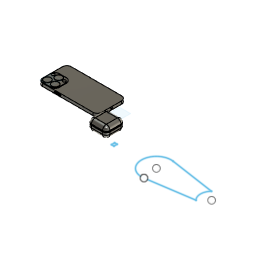
Galaxy Buds v3 (Autodesk Fusion 360 design; units mm, degrees)
Autodesk Fusion 360 part; units mm, degrees
note: some values were not read from the file. Chosen so that the rebuilt part matches the saved one: which bodies a step acts on; which face or edge a step refers to; that a step has no effect.
sketch "Sketch1" plane through (0, 0, 0) normal (0, 0, 1) x (1, 0, 0)
  line L0 (0, 0) -> (50.2, 0)
  line L1 (50.2, 0) -> (50.2, 50)
  line L2 (50.2, 50) -> (0, 50)
  line L3 (0, 50) -> (0, 0)
  dimension "d1" = 50.2
  dimension "d2" = 50
  constraint horizontal L0
  constraint vertical L1
  constraint horizontal L2
  constraint vertical L3
  constraint coincident L0.start L3.end
  measures "d1" distance of L0.start L0.end
  measures "d2" distance of L0.start L2.end
extrude "Extrude1" add sketch "Sketch1" along normal blind 27.88 makes body 1
fillet "Fillet1" radius 10 12 edges at (50.2, 0, 13.94) (25.1, 0, 27.88) (50.2, 25, 27.88) (50.2, 50, 13.94) (50.2, 25, 0) (25.1, 0, 0) (0, 0, 13.94) (0, 25, 27.88) (0, 50, 13.94) (0, 25, 0) (25.1, 50, 0) (25.1, 50, 27.88) on bodies 1
form "Form1" [no effect]
sketch "Sketch2" plane through (0, 0, 0) normal (0, 0, 1) x (1, 0, 0)
  line L0 (0, -10) -> (48, -10)
  line L1 (48, -10) -> (48, -58)
  line L2 (48, -58) -> (0, -58)
  line L3 (0, -58) -> (0, -10)
  dimension "d7" = 48
  dimension "d8" = 48
  constraint horizontal L0
  constraint vertical L1
  constraint horizontal L2
  constraint vertical L3
  measures "d7" distance of L0.start L0.end
  measures "d8" distance of L0.start L2.end
sketch "Sketch3" plane through (0, 0, 0) normal (0, 0, 1) x (1, 0, 0)
  line L0 (150, 0) -> (98.8, 0)
  line L1 (98.8, 0) -> (98.8, 51)
  line L2 (98.8, 51) -> (150, 51)
  line L3 (150, 51) -> (150, 0)
  dimension "d11" = 51.2
  dimension "d12" = 51
  constraint horizontal L0
  constraint vertical L1
  constraint horizontal L2
  constraint vertical L3
  measures "d11" distance of L0.start L0.end
  measures "d12" distance of L0.start L2.end
extrude "Extrude3" add sketch "Sketch3" along normal blind 1 separate body makes body 2
move_body "Move1" bodies 2 to x (1, 0, 0) y (0, 1, 0) z (0, 0, 1) at (-99, 0, 15)
split "Split1" by plane through (-99, 0, 16) normal (0, 0, 1) bodies 1 makes body 3 at (30.1333, 20, 27.88)
move_body "Move2" bodies 3 to x (1, 0, 0) y (0, 1, 0) z (0, 0, 1) at (0, 0, 1)
move_body "Move3" bodies 2 to x (1, 0, 0) y (0, 1, 0) z (0, 0, 1) at (0, 20, 0)
move_body "Move4" bodies 2 to x (1, 0, 0) y (0, 1, 0) z (0, 0, 1) at (0, 100, 0)
sketch "Sketch4" plane through (0, 0, 0) normal (0, 0, 1) x (1, 0, 0)
  line L0 (0, 0) -> (-49.2, 0)
  line L1 (-49.2, 0) -> (-49.2, -49)
  line L2 (-49.2, -49) -> (0, -49)
  line L3 (0, -49) -> (0, 0)
  dimension "d15" = 49.2
  dimension "d16" = 49
  constraint horizontal L0
  constraint vertical L1
  constraint horizontal L2
  constraint vertical L3
  constraint coincident L0.start L3.end
  measures "d15" distance of L0.start L0.end
  measures "d16" distance of L0.start L2.end
extrude "Extrude4" add sketch "Sketch4" along normal blind 1 separate body makes body 4
move_body "Move5" bodies 4 to x (1, 0, 0) y (0, 1, 0) z (0, 0, 1) at (-17, 0, 0)
sketch "Sketch5" plane through (0, 0, 0) normal (0, 1, 0) x (1, 0, 0)
sketch "Sketch6" plane through (0, 0, 1) normal (0, 0, 1) x (-1, 0, 0)
  line L0 (17, 49) -> (17, 0)
  line L1 (17, 0) -> (66.2, 0)
  line L2 (66.2, 0) -> (66.2, 49)
  line L3 (66.2, 49) -> (17, 49)
sketch "Sketch7" plane through (0, 0, 0) normal (0, 0, 1) x (1, 0, 0)
  line L0 (-24.854, -48.854) -> (-17, -48.854)
  line L1 (-17, -48.854) -> (-17, -41)
  line L2 (-17, -41) -> (-24.854, -48.854)
  line L3 (-16.927, -7.781) -> (-16.927, 0.073)
  line L4 (-24.781, 0.073) -> (-16.927, -7.781)
  line L5 (-16.927, 0.073) -> (-24.781, 0.073)
  line L6 (-81.35, 0.006) -> (-89.204, 0.006)
  line L7 (-89.204, -7.848) -> (-81.35, 0.006)
  line L8 (-89.204, 0.006) -> (-89.204, -7.848)
  line L9 (-66.277, -41.067) -> (-66.277, -48.921)
  line L10 (-66.277, -48.921) -> (-58.423, -48.921)
  line L11 (-58.423, -48.921) -> (-66.277, -41.067)
  dimension "d20" = 7.854
  dimension "d21" = 7.854
  dimension "d22" = 7.854
  dimension "d23" = 7.854
  constraint horizontal L0
  constraint vertical L1
  measures "d20" distance of L1.end L0.end
  measures "d21" distance of L4.start L3.end
  measures "d22" distance of L7.start L6.end
  measures "d23" distance of L9.end L10.end
extrude "Extrude5" add sketch "Sketch7" along normal blind 1 separate body contours L6 L7 L8 makes body 5
move_body "Move6" bodies 5 to x (1, 0, 0) y (0, 1, 0) z (0, 0, 1) at (0, 12, 0)
move_body "Move7" bodies 5 to x (1, 0, 0) y (0, 1, 0) z (0, 0, 1) at (23, -12, 0)
split "Split2" by bodies 5 bodies 4 makes body 6 at (-30.7853, -16.3333, 0)
move_body "Move8" bodies 4 to x (1, 0, 0) y (0, 1, 0) z (0, 0, 1) at (0, 9, 0)
extrude "Extrude6" add 1 faces at (-63.5853, 6.3853, 1) along direction (0, 0, 1) blind 1 on bodies 4 bodies 4
move_body "Move9" bodies 4 to x (1, 0, 0) y (0, 1, 0) z (0, 0, 1) at (0, -9, 0)
move_body "Move10" bodies 2 to x (1, 0, 0) y (0, 1, 0) z (0, 0, 1) at (0, -121, 3)
split "Split3" by plane through (-99, -1, 19) normal (0, 0, 1) bodies 3 makes body 7 at (30.1333, 20, 28.88)
move_body "Move11" bodies 3 2 to x (1, 0, 0) y (0, 1, 0) z (0, 0, 1) at (0, 60, 0)
move_body "Move12" bodies 3 to x (1, 0, 0) y (0, 1, 0) z (0, 0, 1) at (137, 0, -11)
scale "Scale1" factor 0.99 about (187.2, 70, 6) bodies 3
move_body "Move13" bodies 3 to x (1, 0, 0) y (0, 1, 0) z (0, 0, 1) at (-138, -60, 10)
move_body "Move14" bodies 3 to x (1, 0, 0) y (0, 1, 0) z (0, 0, 1) at (0.75, 0, 0)
move_body "Move15" bodies 3 to x (1, 0, 0) y (0, 1, 0) z (0, 0, 1) at (0, 0.3, 0)
sketch "Sketch8" plane through (0, 0, 17.98) normal (0, 0, 1) x (-1, 0, 0)
  arc A0 (-40.05, -0.4007) -> (-49.9493, -10.3) centre (-40.05, -10.3) ccw
  line L0 (-49.9493, -10.3) -> (-49.9493, -40)
  arc A1 (-49.9493, -40) -> (-40.05, -49.8993) centre (-40.05, -40) ccw
  line L1 (-40.05, -49.8993) -> (-10.152, -49.8993)
  arc A2 (-10.152, -49.8993) -> (-0.2527, -40) centre (-10.152, -40) ccw
  line L2 (-0.2527, -40) -> (-0.2527, -10.3)
  arc A3 (-0.2527, -10.3) -> (-10.152, -0.4007) centre (-10.152, -10.3) ccw
  line L3 (-10.152, -0.4007) -> (-40.05, -0.4007)
extrude "Extrude7" add sketch "Sketch8" along normal blind 1 bodies 3
move_body "Move16" bodies 2 to x (1, 0, 0) y (0, 1, 0) z (0, 0, 1) at (-94, 0, 0)
sketch "Sketch9" plane through (0, 0, 0) normal (0, 0, 1) x (1, 0, 0)
  line L0 (65, -30) -> (58.35, -30)
  line L1 (58.35, -30) -> (58.35, -21.6)
  line L2 (58.35, -21.6) -> (65, -21.6)
  line L3 (65, -21.6) -> (65, -30)
  dimension "d31" = 6.65
  dimension "d32" = 8.4
  constraint horizontal L0
  constraint vertical L1
  constraint horizontal L2
  constraint vertical L3
  measures "d31" distance of L0.start L0.end
  measures "d32" distance of L0.start L2.end
sketch "Sketch10" plane through (0, 0, 0) normal (1, 0, 0) x (0, 1, 0)
sketch "Sketch11" plane through (0, 0, 0) normal (0, 1, 0) x (1, 0, 0)
  line L0 (44.2, 10) -> (47.545, 10)
  line L1 (44.2, 10) -> (40.855, 10)
  line L2 (44.2, 12.6) -> (40.855, 12.6)
  line L3 (44.2, 12.6) -> (47.545, 12.6)
  arc A0 (47.545, 10) -> (47.545, 12.6) centre (46.9842, 11.3) ccw
  arc A1 (40.855, 12.6) -> (40.855, 10) centre (41.4158, 11.3) ccw
  dimension "d35" = 3.345
  dimension "d36" = 3.345
  dimension "d37" = 3.345
  dimension "d38" = 3.345
  measures "d35" distance of L0.start L0.end
  measures "d36" distance of L0.start L1.end
  measures "d37" distance of L2.start L2.end
  measures "d38" distance of L2.start L3.end
extrude "Extrude8" add sketch "Sketch11" along normal blind 6.65 separate body makes body 8
move_body "Move17" bodies 8 to x (1, 0, 0) y (0, 1, 0) z (0, 0, 1) at (-18, 44, 23)
move_body "Move18" bodies 8 to x (1, 0, 0) y (0, 1, 0) z (0, 0, 1) at (-0.0267, -0.5, -0.4993)
sketch "Sketch12" plane through (0, 0, 0) normal (0, 1, 0) x (1, 0, 0)
split "Split4" by bodies 8 bodies 1 makes body 9 at (20.0667, 16.6667, 16)
move_body "Move19" bodies 8 to x (1, 0, 0) y (0, 1, 0) z (0, 0, 1) at (0, 19, 0)
move_body "Move20" bodies 1 to x (1, 0, 0) y (0, 1, 0) z (0, 0, 1) at (0, 69, 0)
delete_body "RemoveBody1" bodies 1
sketch "Sketch13" plane through (0, 0, 0) normal (0, 1, 0) x (1, 0, 0)
sketch "Sketch14" plane through (0, 0, 0) normal (0, 0, 1) x (1, 0, 0)
  line L0 (-23, 13) -> (-183.6, 13)
  line L1 (-183.6, 13) -> (-183.6, 90.6)
  line L2 (-183.6, 90.6) -> (-23, 90.6)
  line L3 (-23, 90.6) -> (-23, 13)
  dimension "d41" = 160.6
  dimension "d42" = 77.6
  constraint horizontal L0
  constraint vertical L1
  constraint horizontal L2
  constraint vertical L3
  measures "d41" distance of L0.start L0.end
  measures "d42" distance of L0.start L2.end
extrude "Extrude9" add sketch "Sketch14" along normal blind 7.85 separate body makes body 10
fillet "Fillet2" radius 12 4 edges at (-23, 90.6, 3.925) (-23, 13, 3.925) (-183.6, 90.6, 3.925) (-183.6, 13, 3.925) on bodies 10
sketch "Sketch15" plane through (0, 0, 0) normal (0, 0, 1) x (1, 0, 0)
sketch "Sketch16" plane through (0, 0, 0) normal (0, 0, 1) x (1, 0, 0)
  line L0 (0, -25) -> (-30, -25)
  line L1 (-30, -25) -> (-30, 5)
  line L2 (-30, 5) -> (0, 5)
  line L3 (0, 5) -> (0, -25)
  dimension "d47" = 30
  dimension "d48" = 30
  constraint horizontal L0
  constraint vertical L1
  constraint horizontal L2
  constraint vertical L3
  measures "d47" distance of L0.start L0.end
  measures "d48" distance of L0.start L2.end
extrude "Extrude10" add sketch "Sketch16" along normal blind 1 separate body makes body 11
move_body "Move21" bodies 11 to x (1, 0, 0) y (0, 1, 0) z (0, 0, 1) at (-145, 45, 15)
move_body "Move22" bodies 11 to x (1, 0, 0) y (0, 1, 0) z (0, 0, 1) at (0, -8, -3)
move_body "Move23" bodies 11 to x (1, 0, 0) y (0, 1, 0) z (0, 0, 1) at (0, 0, -4)
move_body "Move24" bodies 11 to x (1, 0, 0) y (0, 1, 0) z (0, 0, 1) at (-7, 3, 0)
sketch "Sketch17" plane through (0, 0, 9) normal (0, 0, 1) x (-1, 0, 0)
  line L0 (152, -45) -> (182, -45)
  line L1 (182, -45) -> (182, -15)
  line L2 (182, -15) -> (152, -15)
  line L3 (152, -15) -> (152, -45)
move_body "Move25" bodies 11 to x (1, 0, 0) y (0, 1, 0) z (0, 0, 1) at (-44, 0, 0)
scale "Scale2" factor 1.5 about (-196, 45, 9) bodies 11
move_body "Move26" bodies 11 to x (1, 0, 0) y (0, 1, 0) z (0, 0, 1) at (62, 17, 0)
fillet "Fillet3" radius 12 4 edges at (-179, 17, 8.25) (-134, 17, 8.25) (-134, 62, 8.25) (-179, 62, 8.25) on bodies 11
sketch "Sketch18" plane through (0, 0, 0) normal (0, 0, 1) x (1, 0, 0)
  circle A0 centre (150, 50) radius 9.25
  circle A1 centre (190, 100) radius 9.25
  circle A2 centre (150, 100) radius 9.25
  dimension "d54" = 18.5
  dimension "d55" = 18.5
  dimension "d56" = 18.5
  measures "d54" diameter of A0
  measures "d55" diameter of A1
  measures "d56" diameter of A2
extrude "Extrude11" add sketch "Sketch18" along normal blind 1 separate body contours A0 makes body 12
move_body "Move27" bodies 12 to x (1, 0, 0) y (0, 1, 0) z (0, 0, 1) at (0, 20, 0)
move_body "Move28" bodies 12 to x (1, 0, 0) y (0, 1, 0) z (0, 0, 1) at (-319, -41, 11)
move_body "Move29" bodies 12 to x (1, 0, 0) y (0, 1, 0) z (0, 0, 1) at (0, 0, -2)
copy_body "CopyPasteBodies1" bodies 12 makes body 13
move_body "Move30" bodies 13 to x (1, 0, 0) y (0, 1, 0) z (0, 0, 1) at (11, 22, 0)
move_body "Move31" bodies 12 to x (1, 0, 0) y (0, 1, 0) z (0, 0, 1) at (2, 2, 0)
move_body "Move32" bodies 13 to x (1, 0, 0) y (0, 1, 0) z (0, 0, 1) at (1, 0, 0)
copy_body "CopyPasteBodies2" bodies 13 makes body 14
move_body "Move33" bodies 14 to x (1, 0, 0) y (0, 1, 0) z (0, 0, 1) at (11, -20, 0)
move_body "Move34" bodies 13 to x (1, 0, 0) y (0, 1, 0) z (0, 0, 1) at (1, 0, 0)
sketch "Sketch19" plane through (0, 0, 28.88) normal (0, 0, 1) x (-1, 0, 0)
  line L0 (-40.2, -10) -> (-40.2, -40)
  line L1 (-40.2, -40) -> (-10, -40)
  line L2 (-10, -40) -> (-10, -10)
  line L3 (-10, -10) -> (-40.2, -10)
  circle A0 centre (150, 0) radius 3.9
  dimension "d59" = 7.8
  measures "d59" diameter of A0
extrude "Extrude12" add sketch "Sketch19" along normal blind 0.5 separate body contours A0 makes body 15
move_body "Move35" bodies 15 to x (1, 0, 0) y (0, -1, 0) z (0, 0, -1) at (8, 52, 39.76)
copy_body "CopyPasteBodies3" bodies 15 makes body 16
move_body "Move36" bodies 16 to x (1, 0, 0) y (0, 1, 0) z (0, 0, 1) at (-31, 0, 0)
move_body "Move37" bodies 14 to x (1, 0, 0) y (0, 1, 0) z (0, 0, 1) at (0, -2, 0)
move_body "Move38" bodies 12 to x (1, 0, 0) y (0, 1, 0) z (0, 0, 1) at (0, -2, 0)
move_body "Move39" bodies 13 to x (1, 0, 0) y (0, 1, 0) z (0, 0, 1) at (0, -3, 0)
move_body "Move40" bodies 15 to x (1, 0, 0) y (0, 1, 0) z (0, 0, 1) at (0, -3, 0)
move_body "Move41" bodies 16 to x (1, 0, 0) y (0, 1, 0) z (0, 0, 1) at (0, -4, 0)
scale "Scale3" factor 0.95 about (-146, 62, 9) bodies 11
move_body "Move42" bodies 13 to x (1, 0, 0) y (0, 1, 0) z (0, 0, 1) at (0, 3, 0)
move_body "Move43" bodies 14 to x (1, 0, 0) y (0, 1, 0) z (0, 0, 1) at (0, 2, 0)
move_body "Move44" bodies 12 to x (1, 0, 0) y (0, 1, 0) z (0, 0, 1) at (0, 2, 0)
move_body "Move45" bodies 16 to x (1, 0, 0) y (0, 1, 0) z (0, 0, 1) at (2, 4, 0)
move_body "Move46" bodies 15 to x (1, 0, 0) y (0, 1, 0) z (0, 0, 1) at (0, 2, 0)
move_body "Move47" bodies 16 to x (1, 0, 0) y (0, 1, 0) z (0, 0, 1) at (0, -1, 0)
move_body "Move48" bodies 15 to x (1, 0, 0) y (0, 1, 0) z (0, 0, 1) at (3, 0, 0)
move_body "Move49" bodies 16 to x (1, 0, 0) y (0, 1, 0) z (0, 0, 1) at (1, 0, 0)
move_body "Move50" bodies 16 to x (1, 0, 0) y (0, 1, 0) z (0, 0, 1) at (-1, 0, 0)
move_body "Move51" bodies 15 to x (1, 0, 0) y (0, 1, 0) z (0, 0, 1) at (-2, 0, 0)
move_body "Move52" bodies 15 to x (1, 0, 0) y (0, 1, 0) z (0, 0, 1) at (0, 0, -1)
move_body "Move53" bodies 16 to x (1, 0, 0) y (0, 1, 0) z (0, 0, 1) at (0, 0, -1)
move_body "Move54" bodies 12 to x (1, 0, 0) y (0, 1, 0) z (0, 0, 1) at (1, 0, 0)
move_body "Move55" bodies 12 to x (1, 0, 0) y (0, 1, 0) z (0, 0, 1) at (-0.5, 0, 0)
move_body "Move56" bodies 14 to x (1, 0, 0) y (0, 1, 0) z (0, 0, 1) at (0.5, 0, 0)
move_body "Move57" bodies 11 12 16 13 15 14 to x (1, 0, 0) y (0, 1, 0) z (0, 0, 1) at (-5, -5, 0)
sketch "Sketch20" plane through (0, 0, 28.88) normal (0, 0, 1) x (-1, 0, 0)
  line L0 (-40.2, -10) -> (-40.2, -40)
  line L1 (-40.2, -40) -> (-10, -40)
  line L2 (-10, -40) -> (-10, -10)
  line L3 (-10, -10) -> (-40.2, -10)
sketch "Sketch21" plane through (0, 90.6, 0) normal (0, 1, 0) x (-1, 0, 0)
  line L0 (171.6, 0) -> (171.6, 7.85)
  line L1 (171.6, 7.85) -> (35, 7.85)
  line L2 (35, 7.85) -> (35, 0)
  line L3 (35, 0) -> (171.6, 0)
  arc A0 (36.5, 25) -> (36.5, 22) centre (36.5, 23.5) ccw
  arc A1 (45.1, 22) -> (45.1, 25) centre (45.1, 23.5) ccw
  arc A2 (36.5, 30.5) -> (36.5, 27.5) centre (36.5, 29) ccw
  arc A3 (51.4, 27.5) -> (51.4, 30.5) centre (51.4, 29) ccw
  line L4 (36.5, 30.5) -> (51.4, 30.5)
  line L5 (36.5, 27.5) -> (51.4, 27.5)
  line L6 (36.5, 25) -> (45.1, 25)
  line L7 (36.5, 22) -> (45.1, 22)
  constraint tangent A2 L4
  constraint tangent A3 L5
  constraint tangent A1 L6
  constraint tangent A1 L7
extrude "Extrude13" add sketch "Sketch21" along normal blind 0.5 separate body contours A0 A1 L6 L7 | A2 A3 L4 L5 makes body 17 at (-39.3667, 90.6, 24) makes body 18 at (-41.4667, 90.6, 29.5)
copy_body "CopyPasteBodies4" bodies 17 makes body 19
move_body "Move58" bodies 17 19 to x (1, 0, 0) y (0, 1, 0) z (0, 0, 1) at (-116, 0, -19)
move_body "Move59" bodies 17 to x (1, 0, 0) y (0, 1, 0) z (0, 0, 1) at (0, 0, 3.5)
move_body "Move60" bodies 19 to x (1, 0, 0) y (0, 1, 0) z (0, 0, 1) at (0, 0, -0.5)
move_body "Move61" bodies 17 to x (1, 0, 0) y (0, 1, 0) z (0, 0, 1) at (34, 0, -4)
move_body "Move62" bodies 19 to x (1, 0, 0) y (0, 1, 0) z (0, 0, 1) at (19, 0, 0)
move_body "Move63" bodies 18 to x (1, 0, 0) y (0, 1, 0) z (0, 0, 1) at (-90, -78, -25)
move_body "Move64" bodies 18 to x (1, 0, 0) y (0, 1, 0) z (0, 0, 1) at (3, 0, 0)
sketch "Sketch22" plane through (0, 0, 0) normal (1, 0, 0) x (0, 1, 0)
  arc A0 (116, 7) -> (116, 5) centre (116, 6) ccw
  arc A1 (120.7, 5) -> (120.7, 7) centre (120.7, 6) ccw
  line L0 (116, 7) -> (120.7, 7)
  line L1 (116, 5) -> (120.7, 5)
  constraint tangent A1 L0
  constraint tangent A1 L1
extrude "Extrude14" add sketch "Sketch22" along normal blind 5.7 separate body makes body 20
move_body "Move65" bodies 20 to x (1, 0, 0) y (0, 1, 0) z (0, 0, 1) at (-28.5, -71.5, -1.5)
move_body "Move66" bodies 7 3 9 to x (1, 0, 0) y (0, 1, 0) z (0, 0, 1) at (0, -36.1463, 7.902)
move_body "Move67" bodies 20 to x (1, 0, 0) y (0, 1, 0) z (0, 0, 1) at (0, 4.95, 0)
move_body "Move68" bodies 20 to x (1, 0, 0) y (0, 1, 0) z (0, 0, 1) at (0, 0, -0.574)
split "Split5" by bodies 20 bodies 10 makes body 21 at (-80.5333, 38.8667, 0)
move_body "Move69" bodies 20 to x (1, 0, 0) y (0, 1, 0) z (0, 0, 1) at (19, 0, 0)
sketch "Sketch23" plane through (0, 0, 0) normal (0, 0, 1) x (1, 0, 0)
  line L0 (303.5514, -4.0248) -> (180.9934, 14.5484)
  arc A0 (180.9934, 14.5484) -> (180.9356, -64.5572) centre (175, -25) ccw
  line L1 (303.5514, -45.9752) -> (180.9934, -64.5484)
  arc A1 (303.5514, -4.0248) -> (303.5514, -45.9752) centre (325, -25) ccw
  dimension "d83" = 80
  dimension "d84" = 60
  constraint tangent L0 A0
  measures "d83" diameter of A0
  measures "d84" diameter of A1
hidden bodies 2 4 5 6 8 10 20
equation "d35 = ( 6.69 / 2 ) * 1 mm"
equation "d36 = ( 6.69 / 2 ) * 1 mm"
equation "d37 = ( 6.69 / 2 ) * 1 mm"
equation "d38 = ( 6.69 / 2 ) * 1 mm"
